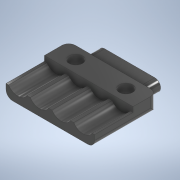
# Autodesk Inventor part: Weight_case_under
Saved by Autodesk Inventor 2020 (Build 240168000, 168)
## iProperties
Created: 2022-06-30
Part Number: Weight_case_under
Material: 一般
Document SubType Name: Modeling
Designer: Masato Kubotera
Density: 1 g/cm^3
Appearance: 濃い灰色
Author: Masato Kubotera
Autodesk Inventor part; units mm, degrees
ref_plane "YZ Plane" through (0, 0, 0) normal (1, 0, 0) x (0, 1, 0)
ref_plane "XZ Plane" through (0, 0, 0) normal (0, 1, 0) x (-1, 0, 0)
ref_plane "XY Plane" through (0, 0, 0) normal (0, 0, 1) x (1, 0, 0)
sketch "スケッチ1" plane through (0, 0, 0) normal (1, 0, 0) x (0, 1, 0)
  arc A0 (-7.5, 1.25) -> (-7.5, -2.75) centre (-7.5, -0.75) ccw construction
  line L0 (-7.5, 1.25) -> (7.5, 1.25) construction
  line L1 (0, 2.5) -> (0, -2.5) construction
  arc A1 (7.5, -2.75) -> (7.5, 1.25) centre (7.5, -0.75) ccw construction
  arc A2 (-7.5, 1) -> (-7.5, -2.5) centre (-7.5, -0.75) ccw
  line L2 (-7.5, 1) -> (7.5, 1)
  line L3 (-7.5, -2.5) -> (7.5, -2.5)
  arc A3 (7.5, -2.5) -> (7.5, 1) centre (7.5, -0.75) ccw
  line L4 (-7.5, -2.75) -> (7.5, -2.75) construction
  line L5 (-13.5, 2.5) -> (13.5, 2.5) construction
  line L6 (13.5, 2.5) -> (13.5, -2.5) construction
  line L7 (13.5, -2.5) -> (-13.5, -2.5) construction
  line L8 (-13.5, -2.5) -> (-13.5, 2.5) construction
  line L9 (-13.5, 2.5) -> (13.5, -2.5) construction
  line L10 (13.5, 2.5) -> (-13.5, -2.5) construction
  line L11 (-13.25, 2.5) -> (13.25, 2.5)
  line L12 (13.25, 2.5) -> (13.25, -2.5)
  line L13 (13.25, -2.5) -> (-13.25, -2.5)
  line L14 (-13.25, -2.5) -> (-13.25, 2.5)
  line L15 (-13.25, 2.5) -> (13.25, -2.5) construction
  line L16 (13.25, 2.5) -> (-13.25, -2.5) construction
  circle A4 centre (-9.75, 2.75) radius 3.25 construction
  circle A5 centre (-3.25, 2.75) radius 3.25 construction
  circle A6 centre (3.25, 2.75) radius 3.25 construction
  circle A7 centre (9.75, 2.75) radius 3.25 construction
  arc A8 (-5.9886, 1) -> (-0.5114, 1) centre (-3.25, 2.75) ccw
  arc A9 (0.5114, 1) -> (5.9886, 1) centre (3.25, 2.75) ccw
  line L17 (-9.75, 2.75) -> (9.75, 2.75) construction
  line L18 (0, 2.5) -> (0, -2.75) construction
  line L19 (-7.0114, 1) -> (-5.9886, 1)
  line L20 (-0.5114, 1) -> (0.5114, 1)
  line L21 (5.9886, 1) -> (7.0114, 1)
  line L22 (-12.4886, 1) -> (-13.25, 1)
  line L23 (12.4886, 1) -> (13.25, 1)
  arc A10 (-12.9904, 2.5) -> (-12.9815, 2.404) centre (-9.75, 2.75) ccw
  arc A11 (-12.4886, 1) -> (-7.0114, 1) centre (-9.75, 2.75) ccw
  arc A12 (7.0114, 1) -> (12.4886, 1) centre (9.75, 2.75) ccw
  arc A13 (12.9815, 2.404) -> (12.9904, 2.5) centre (9.75, 2.75) ccw
  point P0 (0, 0)
  point P1 (0, 0)
  point P2 (0, 0)
  point P3 (-0.0096, 2.5)
  point P4 (0.0096, 2.5)
  point P5 (6.4904, 2.5)
  point P6 (0, 2.75)
  point P7 (-7.5, -2.5)
  point P8 (5.9886, 1)
  point P9 (0.5114, 1)
  point P10 (-0.5114, 1)
  point P11 (-5.9886, 1)
  point P12 (-6.9904, 2.5)
  point P13 (-7.0114, 1)
  point P14 (9.2254, -0.4574)
  point P15 (7.0114, 1)
  point P16 (-7.5, -2.5)
  point P17 (-9.2254, -0.4574)
  point P18 (-7.0114, 1)
  dimension "d0" = 2
  dimension "d1" = 15
  dimension "d2" = 0.25
  dimension "d3" = 6
  dimension "d4" = 6
  dimension "d5" = 0.25
  dimension "d6" = 5
  dimension "d7" = 6.5
  dimension "d8" = 6.5
  dimension "d10" = 6.5
  dimension "d12" = 6.5
  dimension "d27" = 1.5
  dimension "d28" = 2
  dimension "d29" = 0.7614
  constraints: 46 end point, 31 point on circle, 14 centre point, 12 point on line, 10 tangent, 9 midpoint, 7 coincident, 7 horizontal, 4 collinear, 3 parallel, 3 perpendicular, 2 concentric, 1 vertical, 11 other
  measures "d0" radius of A0
  measures "d1" distance of L0.start L0.end
  measures "d2" radial gap between concentric circles of A0 A2
  measures "d3" horizontal distance of L7.end A0.centre
  measures "d4" horizontal distance of L6.end A1.centre
  measures "d5" distance between parallel lines of L8 L14
  measures "d6" distance of L12.start L12.end
  measures "d7" diameter of A4
  measures "d8" diameter of A5
  measures "d10" diameter of A6
  measures "d12" diameter of A7
  measures "d28" distance edge to line of A4 L13
  measures "d29" distance of L22.start L22.end
extrude "押し出し1" add sketch "スケッチ1" against normal blind 33.75 contours L2 A11 A2 | A11 L2 A8 A9 A12 A3 L3 A2 | L2 A8 | A12 L2 A3 | L2 A9
extrude "押し出し2" add sketch "スケッチ1" against normal blind 28.75
extrude "押し出し3" cut sketch "スケッチ1" against normal blind 21.5 contours L2 A11 A2 | A2 A11 L22 L14 L11 L12 L23 A12 A3 L2 | L2 A8 | A12 L2 A3 | L2 A9
extrude "押し出し4" cut sketch "スケッチ1" against normal blind 10
sketch "スケッチ2" plane through (-28.75, -13.25, 2.5) normal (0, 0, 1) x (1, 0, 0)
  line L0 (0, 0) -> (0, 26.5) projected
  line L1 (18.75, 26.5) -> (0, 26.5) projected
  line L2 (0, 0) -> (7.25, 0)
  line L3 (7.25, 0) -> (7.25, 26.5)
  line L4 (7.25, 26.5) -> (0, 26.5)
  line L5 (0, 26.5) -> (0, 0)
  line L6 (7.25, 0) -> (7.25, 26.5) projected
  line L7 (18.75, 0) -> (0, 0) projected
  line L8 (3.625, 0) -> (3.625, 26.5) construction
  line L9 (18.75, 26.5) -> (0, 26.5) projected
  circle A0 centre (3.625, 5.75) radius 2
  line L10 (0, 13.25) -> (7.25, 13.25) construction
  circle A1 centre (3.625, 20.75) radius 2
  point P0 (28.75, 13.25)
  point P1 (7.25, 0.2596)
  point P2 (7.25, 7.2404)
  point P3 (7.25, 26.2404)
  dimension "d23" = 4
  dimension "d24" = 15
  constraints: 12 end point, 4 point on line, 3 midpoint, 3 parallel, 2 centre point, 2 perpendicular, 1 collinear, 1 horizontal, 1 symmetric about line, 1 other
  measures "d23" diameter of A0
  measures "d24" distance of A1.centre A0.centre
extrude "押し出し5" cut sketch "スケッチ2" against normal through all contours A0 | A1
fillet "フィレット1" radius 2 4 edges at (-28.75, -13.25, 0) (-28.75, 13.25, 0) (-19.375, 13.25, -2.5) (-19.375, -13.25, -2.5)
equation "\"d5\" = d2"
